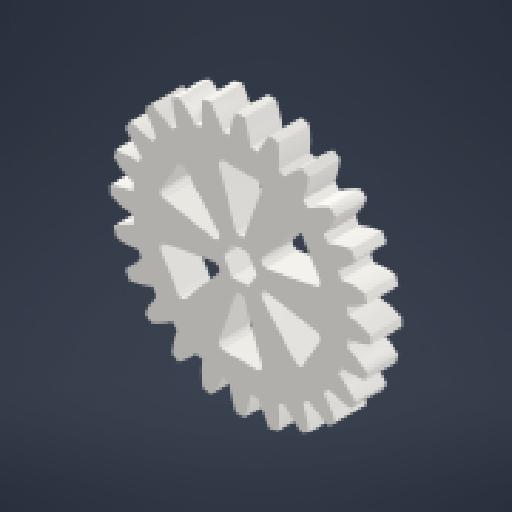
# Autodesk Inventor part: Spur Gear2
Saved by Autodesk Inventor 2023 (Build 270158000, 158)
## iProperties
CustomPartVersion: 1
Created: 2022-11-20
Part Number: Spur Gear2
Material: Steel
Document SubType Name: Modeling
Designer: Izack Waczko
Categories: <?xml version="1.0" encoding="UTF-16"?> <MemberInstance><Categories><FamilyTemplate><FamilyTemplateParameter ValueType="xs:double" Id="1" ObjectReferenceKey="da_z" ObjectType="kUserParameterObject"/><FamilyTemplateParameter ValueType="xs:double" Id="2" ObjectReferenceKey="da_b" ObjectType="kUserParameterObject"/><FamilyTemplateParameter ValueType="xs:double" Id="3" ObjectReferenceKey="da_beta" ObjectType="kUserParameterObject"/><FamilyTemplateParameter ValueType="xs:double" Id="4" ObjectReferenceKey="da_da" ObjectType="kUserParameterObject"/><FamilyTemplateParameter ValueType="xs:double" Id="5" ObjectReferenceKey="da_aw" ObjectType="kUserParameterObject"/><FamilyTemplateParameter ValueType="xs:string" Id="6" ObjectReferenceKey="EAIAABAAAACIAQAAAAAAAIAAAAAAAAAA" ObjectType="83910656" SubObjectId="SurfaceGeometry"/></FamilyTemplate><ParamToTemplateMap><ParamToTemplate CategoryParameter="//CategoryParameter[@InternalName='046C89C9-8512-4d59-83FE-43B91F4F132A']" TemplateParameter="1"/><ParamToTemplate CategoryParameter="//CategoryParameter[@InternalName='2552DF32-E462-4b46-AEBF-C6C7768E72AC']" TemplateParameter="2"/><ParamToTemplate CategoryParameter="//CategoryParameter[@InternalName='C9EE641D-15FC-4fae-A226-E94C4372FDD7']" TemplateParameter="3"/><ParamToTemplate><ParamToTemplate CategoryParameter="//CategoryParameter[@InternalName='00B6519A-459B-49c7-AD84-2E56D39A5744']" ConstantValue="0.204114"/></ParamToTemplate><ParamToTemplate><ParamToTemplate CategoryParameter="//CategoryParameter[@InternalName='04B31F0E-C7A6-4894-AA32-9629BEFACF47']" ConstantValue="1.000000"/></ParamToTemplate><ParamToTemplate><ParamToTemplate CategoryParameter="//CategoryParameter[@InternalName='43CBEC2E-7847-49e7-A936-2F7889FCB2D9']" ConstantValue="0.250000"/></ParamToTemplate><ParamToTemplate><ParamToTemplate CategoryParameter="//CategoryParameter[@InternalName='B1EFC894-105D-4ebd-86BF-FA20ED196853']" ConstantValue="0.350000"/></ParamToTemplate><ParamToTemplate><ParamToTemplate CategoryParameter="//CategoryParameter[@InternalName='51175063-3D10-4879-93E8-6246FE8B403D']" ConstantValue="2060000000.000000"/></ParamToTemplate><ParamToTemplate><ParamToTemplate CategoryParameter="//CategoryParameter[@InternalName='A3A52E27-4454-46a9-B0BD-C932399B70AF']" ConstantValue="0.300000"/></ParamToTemplate><ParamToTemplate><ParamToTemplate CategoryParameter="//CategoryParameter[@InternalName='91B76062-C214-41d9-B1B9-14D2AB99603D']" ConstantValue="0.250000"/></ParamToTemplate><ParamToTemplate><ParamToTemplate CategoryParameter="//CategoryParameter[@InternalName='374E806E-8B8A-4dda-A9AA-1039D6500AD2']" ConstantValue="4.000000"/></ParamToTemplate><ParamToTemplate><ParamToTemplate CategoryParameter="//CategoryParameter[@InternalName='2D373A89-B862-43d6-8D0B-0CBF12AB9F6C']" ConstantValue="0.349066"/></ParamToTemplate><ParamToTemplate CategoryParameter="//CategoryParameter[@InternalName='37777632-D6A2-4fac-9D53-DB8ACD95C989']" TemplateParameter="4"/><ParamToTemplate CategoryParameter="//CategoryParameter[@InternalName='FD1017F1-B727-4f7e-9707-0F86F1FF9423']" TemplateParameter="5"/><ParamToTemplate><ParamToTemplate CategoryParameter="//CategoryParameter[@InternalName='9E1B4470-B2D3-4ff1-B813-535BB4CDF51A']" ConstantValue="3520000.000000"/></ParamToTemplate><ParamToTemplate><ParamToTemplate CategoryParameter="//CategoryParameter[@InternalName='F8452263-BFF6-458c-9FB1-07C4B99E95CD']" ConstantValue="11400000.000000"/></ParamToTemplate><ParamToTemplate><ParamToTemplate CategoryParameter="//CategoryParameter[@InternalName='3E3BB259-FD49-497f-8171-6EBC954A3479']" ConstantValue="2.000000"/></ParamToTemplate><ParamToTemplate CategoryParameter="//CategoryParameter[@InternalName='27C3BAF2-7550-4e4b-AE2C-0DB134B7D9B7']" TemplateParameter="6"/></ParamToTemplateMap><Category DisplayName="Gear" InternalName="DC85795E-93AB-48d5-8EEE-5A27447B64BD" Mnemonic="Gear"><CategoryParameter DisplayName="z" InternalName="046C89C9-8512-4d59-83FE-43B91F4F132A" Mnemonic="z"/><CategoryParameter DisplayName="b" InternalName="2552DF32-E462-4b46-AEBF-C6C7768E72AC" Mnemonic="b"/><CategoryParameter DisplayName="||b|" InternalName="C9EE641D-15FC-4fae-A226-E94C4372FDD7" Mnemonic="beta"/><CategoryParameter DisplayName="x" InternalName="00B6519A-459B-49c7-AD84-2E56D39A5744" Mnemonic="x"/><CategoryParameter DisplayName="a*" InternalName="04B31F0E-C7A6-4894-AA32-9629BEFACF47" Mnemonic="a"/><CategoryParameter DisplayName="c*" InternalName="43CBEC2E-7847-49e7-A936-2F7889FCB2D9" Mnemonic="c"/><CategoryParameter DisplayName="r|.f|*" InternalName="B1EFC894-105D-4ebd-86BF-FA20ED196853" Mnemonic="rf"/><CategoryParameter DisplayName="E" InternalName="51175063-3D10-4879-93E8-6246FE8B403D" Mnemonic="E"/><CategoryParameter DisplayName="||m|" InternalName="A3A52E27-4454-46a9-B0BD-C932399B70AF" Mnemonic="mi"/><Category DisplayName="SpurGear" InternalName="26C5A22E-A91E-4dfd-A3B3-23CCAFAE1764" Mnemonic="SpurGear"><CategoryParameter DisplayName="m" InternalName="91B76062-C214-41d9-B1B9-14D2AB99603D" Mnemonic="m"/><CategoryParameter DisplayName="P" InternalName="374E806E-8B8A-4dda-A9AA-1039D6500AD2" Mnemonic="PP"/><CategoryParameter DisplayName="||a|" InternalName="2D373A89-B862-43d6-8D0B-0CBF12AB9F6C" Mnemonic="alpha"/><CategoryParameter DisplayName="d|.a|" InternalName="37777632-D6A2-4fac-9D53-DB8ACD95C989" Mnemonic="da"/><CategoryParameter DisplayName="a|.w|" InternalName="FD1017F1-B727-4f7e-9707-0F86F1FF9423" Mnemonic="aw"/><CategoryParameter DisplayName="||s||.Flim|" InternalName="9E1B4470-B2D3-4ff1-B813-535BB4CDF51A" Mnemonic="sFlim"/><CategoryParameter DisplayName="||s||.Hlim|" InternalName="F8452263-BFF6-458c-9FB1-07C4B99E95CD" Mnemonic="sHlim"/><CategoryParameter DisplayName="type" InternalName="3E3BB259-FD49-497f-8171-6EBC954A3479" Mnemonic="type"/><CategoryParameter DisplayName="PitchDiameter" InternalName="27C3BAF2-7550-4e4b-AE2C-0DB134B7D9B7" Mnemonic="IDS_PITCHDIAM"/></Category></Category></Categories></MemberInstance>
Density: 1 g/cm^3
Appearance: Steel
Author: Izack Waczko
Autodesk Inventor part; units mm, degrees
sketch "Sketch1" plane through (0, 0, 0) normal (0, 0, 1) x (1, 0, 0)
  circle A0 centre (0, 0) radius 33
  dimension "d0" = 66
  constraints: 1 centre point
  measures "d0" diameter of A0
extrude "Extrusion1" add sketch "Sketch1" along normal blind 8
ref_plane "Work Plane2" through (0, 0, 4) normal (0, 0, 1) x (1, 0, 0)
sketch "Sketch2" plane through (0, 0, 0) normal (0, 0, -1) x (-1, 0, 0)
  circle A0 centre (0, 0) radius 33 projected
  circle A1 centre (0, 0) radius 30
  dimension "d3" = 60
  constraints: 1 centre point, 1 coincident
  measures "d3" diameter of A1
surface extrude "Pitch Diameter" sketch "Sketch2" against normal through all shown no curves A1
ref_plane "Work Plane8" through (0, 0, 0) normal (0.9914449, 0.1305262, 0) x (0, 0, 1)
ref_plane "Work Plane9" through (0, 0, 0) normal (1, 0, 0) x (0, 1, 0)
spur gear teeth "Spur Gear" teeth 24 pitch diameter 60 tip diameter 66 root diameter 54.7706 face width 8 start plane through (0, 0, 0) normal (0, 0, -1) x (-1, 0, 0)
sketch "Sketch3" plane through (0, 0, 8) normal (0, 0, 1) x (1, 0, 0)
  circle A0 centre (0, 0) radius 3.65 construction
  line L0 (2.1073, 3.65) -> (4.2147, 0)
  line L1 (4.2147, 0) -> (2.1073, -3.65)
  line L2 (2.1073, -3.65) -> (-2.1073, -3.65)
  line L3 (-2.1073, -3.65) -> (-4.2147, 0)
  line L4 (-4.2147, 0) -> (-2.1073, 3.65)
  line L5 (-2.1073, 3.65) -> (2.1073, 3.65)
  circle A1 centre (0, 0) radius 7.5 construction
  circle A2 centre (0, 0) radius 20 construction
  arc A3 (1.1799, -7.0873) -> (-1.1799, -7.0873) centre (0, -7.5) ccw
  arc A4 (4.2147, -20.8009) -> (5.3946, -19.1382) centre (4.2147, -19.5509) ccw
  arc A5 (-5.3946, -19.1382) -> (-4.2147, -20.8009) centre (-4.2147, -19.5509) ccw
  line L6 (1.1799, -7.0873) -> (5.433, -19.2479)
  line L7 (4.2147, -20.8009) -> (-4.2147, -20.8009)
  line L8 (-5.433, -19.2479) -> (-1.1799, -7.0873)
  arc A6 (20.1214, -6.7504) -> (19.2715, -4.8973) centre (19.0389, -6.1254) ccw
  line L9 (20.1214, -6.7504) -> (15.9068, -14.0504)
  arc A7 (13.8769, -14.2409) -> (15.9068, -14.0504) centre (14.8242, -13.4254) ccw
  line L10 (13.9527, -14.329) -> (5.5479, -4.5655)
  arc A8 (6.7278, -2.5218) -> (5.5479, -4.5655) centre (6.4952, -3.75) ccw
  line L11 (6.7278, -2.5218) -> (19.3857, -4.9189)
  arc A9 (15.9068, 14.0504) -> (13.8769, 14.2409) centre (14.8242, 13.4254) ccw
  line L12 (15.9068, 14.0504) -> (20.1214, 6.7504)
  arc A10 (19.2715, 4.8973) -> (20.1214, 6.7504) centre (19.0389, 6.1254) ccw
  line L13 (19.3857, 4.9189) -> (6.7278, 2.5218)
  arc A11 (5.5479, 4.5655) -> (6.7278, 2.5218) centre (6.4952, 3.75) ccw
  line L14 (5.5479, 4.5655) -> (13.9527, 14.329)
  arc A12 (-4.2147, 20.8009) -> (-5.3946, 19.1382) centre (-4.2147, 19.5509) ccw
  line L15 (-4.2147, 20.8009) -> (4.2147, 20.8009)
  arc A13 (5.3946, 19.1382) -> (4.2147, 20.8009) centre (4.2147, 19.5509) ccw
  line L16 (5.433, 19.2479) -> (1.1799, 7.0873)
  arc A14 (-1.1799, 7.0873) -> (1.1799, 7.0873) centre (0, 7.5) ccw
  line L17 (-1.1799, 7.0873) -> (-5.433, 19.2479)
  arc A15 (-20.1214, 6.7504) -> (-19.2715, 4.8973) centre (-19.0389, 6.1254) ccw
  line L18 (-20.1214, 6.7504) -> (-15.9068, 14.0504)
  arc A16 (-13.8769, 14.2409) -> (-15.9068, 14.0504) centre (-14.8242, 13.4254) ccw
  line L19 (-13.9527, 14.329) -> (-5.5479, 4.5655)
  arc A17 (-6.7278, 2.5218) -> (-5.5479, 4.5655) centre (-6.4952, 3.75) ccw
  line L20 (-6.7278, 2.5218) -> (-19.3857, 4.9189)
  arc A18 (-15.9068, -14.0504) -> (-13.8769, -14.2409) centre (-14.8242, -13.4254) ccw
  line L21 (-15.9068, -14.0504) -> (-20.1214, -6.7504)
  arc A19 (-19.2715, -4.8973) -> (-20.1214, -6.7504) centre (-19.0389, -6.1254) ccw
  line L22 (-19.3857, -4.9189) -> (-6.7278, -2.5218)
  arc A20 (-5.5479, -4.5655) -> (-6.7278, -2.5218) centre (-6.4952, -3.75) ccw
  line L23 (-5.5479, -4.5655) -> (-13.9527, -14.329)
  point P0 (0, 3.65)
  dimension "d49" = 7.3
  dimension "d52" = 15
  dimension "d53" = 40
  dimension "d54" = 2.5
  dimension "d55" = 2.5
  dimension "d56" = 2.5
  dimension "d59" = 360
  constraints: 48 end point, 40 point on circle, 19 centre point, 12 point on line, 6 tangent, 4 coincident, 2 vertical alignment, 1 horizontal, 1 midpoint, 120 other
  measures "d53" diameter of A2
  measures "d54" diameter of A3
  measures "d55" diameter of A4
  measures "d56" diameter of A5
extrude "Extrusion2" cut sketch "Sketch3" against normal up to surface (8 mm away)
equation "\"d0\" = da_da"
equation "\"d1\" = da_b"
equation "\"d3\" = da_d"
equation "\"d16\" = da_aw"
equation "\"d43\" = da_aw"
equation "\"d46\" = da_aw"
equation "\"da_da\" = 66"
equation "\"da_b\" = 8"
equation "\"da_d\" = 60"
equation "\"da_aw\" = 90.5"
body "Solid1"
body "Srf1"
